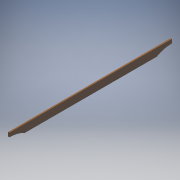
# Autodesk Inventor part: Support Beam
Saved by Autodesk Inventor 2016 (Build 200138000, 138)
## iProperties
Created: 2014-06-08
Part Number: Support Beam
Material: Generic
Document SubType Name: Modeling
Designer: Haden
Density: 1 g/cm^3
Appearance: Default
Author: Haden
Autodesk Inventor part; units mm, degrees
ref_plane "YZ Plane" through (0, 0, 0) normal (1, 0, 0) x (0, 1, 0)
ref_plane "XZ Plane" through (0, 0, 0) normal (0, 1, 0) x (-1, 0, 0)
ref_plane "XY Plane" through (0, 0, 0) normal (0, 0, 1) x (1, 0, 0)
sketch "Sketch1" plane through (0, 0, 0) normal (0, 0, 1) x (1, 0, 0)
  line L0 (0, 0) -> (38.1, 0)
  line L1 (38.1, 0) -> (38.1, -234.95)
  line L2 (38.1, -234.95) -> (0, -234.95)
  line L3 (0, -234.95) -> (0, 0)
  dimension "d0" = 38.1
  dimension "d1" = 234.95
  constraints: 8 end point, 2 parallel, 1 horizontal, 1 perpendicular
  measures "d0" distance of L1.end L2.end
  measures "d1" distance of L0.end L1.end
extrude "Extrusion1" add sketch "Sketch1" along normal blind 4876.8
sketch "Sketch2" plane through (38.1, -234.95, 0) normal (1, 0, 0) x (0, 0, -1)
  line L0 (0, 234.95) -> (0, 0) projected
  line L1 (0, 234.95) -> (-4876.8, 234.95) projected
  line L2 (-4876.8, 0) -> (-4876.8, 234.95) projected
  line L3 (0, 0) -> (-4876.8, 0) projected
  line L4 (0, 0) -> (0, 234.95) projected
  arc A0 (0, 117.475) -> (-457.2, 0) centre (0, -830.949) ccw
  arc A1 (-4419.6, 0) -> (-4876.8, 117.475) centre (-4876.8, -830.949) ccw
  line L5 (-4876.8, 0) -> (-4876.8, 234.95) construction
  dimension "d7" = 457.2
  dimension "d8" = 457.2
  constraints: 4 midpoint, 4 point on circle, 4 point on line, 2 centre point
  measures "d7" distance from line of L0 A0.end
  measures "d8" distance from line of A1.start L2
extrude "Extrusion2" cut sketch "Sketch2" along normal through all both and the other way through all contours L0 L3 A0 | A1 L3 L2
body "Solid1"
